Autodesk Fusion 360 part; units mm, degrees
(part 5 of 6)
  line L1119 (10, 7.0711) -> (7.0711, 10)
  line L1120 (7.0711, 10) -> (10, 12.9289)
  line L1121 (10, 12.9289) -> (12.9289, 10)
  line L1122 (12.9289, -10) -> (10, -12.9289)
  line L1123 (10, -12.9289) -> (7.0711, -10)
  line L1124 (7.0711, -10) -> (10, -7.0711)
  line L1125 (10, -7.0711) -> (12.9289, -10)
  line L1126 (2.9289, 10) -> (0, 7.0711)
  line L1127 (0, 7.0711) -> (-2.9289, 10)
  line L1128 (-2.9289, 10) -> (0, 12.9289)
  line L1129 (0, 12.9289) -> (2.9289, 10)
  line L1130 (12.9289, 0) -> (10, -2.9289)
  line L1131 (10, -2.9289) -> (7.0711, 0)
  line L1132 (7.0711, 0) -> (10, 2.9289)
  line L1133 (10, 2.9289) -> (12.9289, 0)
  line L1134 (2.9289, 0) -> (0, -2.9289)
  line L1135 (0, -2.9289) -> (-2.9289, 0)
  line L1136 (-2.9289, 0) -> (0, 2.9289)
  line L1137 (0, 2.9289) -> (2.9289, 0)
  line L1138 (2.9289, -10) -> (0, -12.9289)
  line L1139 (0, -12.9289) -> (-2.9289, -10)
  line L1140 (-2.9289, -10) -> (0, -7.0711)
  line L1141 (0, -7.0711) -> (2.9289, -10)
  line L1142 (2.9289, 40) -> (0, 37.0711)
  line L1143 (0, 37.0711) -> (-2.9289, 40)
  line L1144 (-2.9289, 40) -> (0, 42.9289)
  line L1145 (0, 42.9289) -> (2.9289, 40)
  line L1146 (42.9289, 20) -> (40, 17.0711)
  line L1147 (40, 17.0711) -> (37.0711, 20)
  line L1148 (37.0711, 20) -> (40, 22.9289)
  line L1149 (40, 22.9289) -> (42.9289, 20)
  line L1150 (-7.0711, 40) -> (-10, 37.0711)
  line L1151 (-10, 37.0711) -> (-12.9289, 40)
  line L1152 (-12.9289, 40) -> (-10, 42.9289)
  line L1153 (-10, 42.9289) -> (-7.0711, 40)
  line L1154 (42.9289, 10) -> (40, 7.0711)
  line L1155 (40, 7.0711) -> (37.0711, 10)
  line L1156 (37.0711, 10) -> (40, 12.9289)
  line L1157 (40, 12.9289) -> (42.9289, 10)
  line L1158 (42.9289, 0) -> (40, -2.9289)
  line L1159 (40, -2.9289) -> (37.0711, 0)
  line L1160 (37.0711, 0) -> (40, 2.9289)
  line L1161 (40, 2.9289) -> (42.9289, 0)
  line L1162 (42.9289, -10) -> (40, -12.9289)
  line L1163 (40, -12.9289) -> (37.0711, -10)
  line L1164 (37.0711, -10) -> (40, -7.0711)
  line L1165 (40, -7.0711) -> (42.9289, -10)
  line L1166 (42.9289, -20) -> (40, -22.9289)
  line L1167 (40, -22.9289) -> (37.0711, -20)
  line L1168 (37.0711, -20) -> (40, -17.0711)
  line L1169 (40, -17.0711) -> (42.9289, -20)
  line L1170 (42.9289, -30) -> (40, -32.9289)
  line L1171 (40, -32.9289) -> (37.0711, -30)
  line L1172 (37.0711, -30) -> (40, -27.0711)
  line L1173 (40, -27.0711) -> (42.9289, -30)
  line L1174 (42.9289, -40) -> (40, -42.9289)
  line L1175 (40, -42.9289) -> (37.0711, -40)
  line L1176 (37.0711, -40) -> (40, -37.0711)
  line L1177 (40, -37.0711) -> (42.9289, -40)
  line L1178 (32.9289, -40) -> (30, -42.9289)
  line L1179 (30, -42.9289) -> (27.0711, -40)
  line L1180 (27.0711, -40) -> (30, -37.0711)
  line L1181 (30, -37.0711) -> (32.9289, -40)
  line L1182 (22.9289, -40) -> (20, -42.9289)
  line L1183 (20, -42.9289) -> (17.0711, -40)
  line L1184 (17.0711, -40) -> (20, -37.0711)
  line L1185 (20, -37.0711) -> (22.9289, -40)
  line L1186 (12.9289, -40) -> (10, -42.9289)
  line L1187 (10, -42.9289) -> (7.0711, -40)
  line L1188 (7.0711, -40) -> (10, -37.0711)
  line L1189 (10, -37.0711) -> (12.9289, -40)
  line L1190 (2.9289, -40) -> (0, -42.9289)
  line L1191 (0, -42.9289) -> (-2.9289, -40)
  line L1192 (-2.9289, -40) -> (0, -37.0711)
  line L1193 (0, -37.0711) -> (2.9289, -40)
  line L1194 (-7.0711, -40) -> (-10, -42.9289)
  line L1195 (-10, -42.9289) -> (-12.9289, -40)
  line L1196 (-12.9289, -40) -> (-10, -37.0711)
  line L1197 (-10, -37.0711) -> (-7.0711, -40)
  line L1198 (-17.0711, -30) -> (-20, -32.9289)
  line L1199 (-20, -32.9289) -> (-22.9289, -30)
  line L1200 (-22.9289, -30) -> (-20, -27.0711)
  line L1201 (-20, -27.0711) -> (-17.0711, -30)
  line L1202 (-27.0711, -30) -> (-30, -32.9289)
  line L1203 (-30, -32.9289) -> (-32.9289, -30)
  line L1204 (-32.9289, -30) -> (-30, -27.0711)
  line L1205 (-30, -27.0711) -> (-27.0711, -30)
  line L1206 (-37.0711, -40) -> (-40, -42.9289)
  line L1207 (-40, -42.9289) -> (-42.9289, -40)
  line L1208 (-42.9289, -40) -> (-40, -37.0711)
  line L1209 (-40, -37.0711) -> (-37.0711, -40)
  line L1210 (-47.0711, -50) -> (-50, -52.9289)
  line L1211 (-50, -52.9289) -> (-52.9289, -50)
  line L1212 (-52.9289, -50) -> (-50, -47.0711)
  line L1213 (-50, -47.0711) -> (-47.0711, -50)
  line L1214 (-47.0711, -40) -> (-50, -42.9289)
  line L1215 (-50, -42.9289) -> (-52.9289, -40)
  line L1216 (-52.9289, -40) -> (-50, -37.0711)
  line L1217 (-50, -37.0711) -> (-47.0711, -40)
  line L1218 (-47.0711, -30) -> (-50, -32.9289)
  line L1219 (-50, -32.9289) -> (-52.9289, -30)
  line L1220 (-52.9289, -30) -> (-50, -27.0711)
  line L1221 (-50, -27.0711) -> (-47.0711, -30)
  line L1222 (-47.0711, -20) -> (-50, -22.9289)
  line L1223 (-50, -22.9289) -> (-52.9289, -20)
  line L1224 (-52.9289, -20) -> (-50, -17.0711)
  line L1225 (-50, -17.0711) -> (-47.0711, -20)
  line L1226 (-47.0711, -10) -> (-50, -12.9289)
  line L1227 (-50, -12.9289) -> (-52.9289, -10)
  line L1228 (-52.9289, -10) -> (-50, -7.0711)
  line L1229 (-50, -7.0711) -> (-47.0711, -10)
  line L1230 (-47.0711, 0) -> (-50, -2.9289)
  line L1231 (-50, -2.9289) -> (-52.9289, 0)
  line L1232 (-52.9289, 0) -> (-50, 2.9289)
  line L1233 (-50, 2.9289) -> (-47.0711, 0)
  line L1234 (-47.0711, 30) -> (-50, 27.0711)
  line L1235 (-50, 27.0711) -> (-52.9289, 30)
  line L1236 (-52.9289, 30) -> (-50, 32.9289)
  line L1237 (-50, 32.9289) -> (-47.0711, 30)
  line L1238 (-17.0711, -40) -> (-20, -42.9289)
  line L1239 (-20, -42.9289) -> (-22.9289, -40)
  line L1240 (-22.9289, -40) -> (-20, -37.0711)
  line L1241 (-20, -37.0711) -> (-17.0711, -40)
  line L1242 (22.9289, -50) -> (20, -52.9289)
  line L1243 (20, -52.9289) -> (17.0711, -50)
  line L1244 (17.0711, -50) -> (20, -47.0711)
  line L1245 (20, -47.0711) -> (22.9289, -50)
  line L1246 (52.9289, -40) -> (50, -42.9289)
  line L1247 (50, -42.9289) -> (47.0711, -40)
  line L1248 (47.0711, -40) -> (50, -37.0711)
  line L1249 (50, -37.0711) -> (52.9289, -40)
  line L1250 (52.9289, -50) -> (50, -52.9289)
  line L1251 (50, -52.9289) -> (47.0711, -50)
  line L1252 (47.0711, -50) -> (50, -47.0711)
  line L1253 (50, -47.0711) -> (52.9289, -50)
  line L1254 (32.9289, -50) -> (30, -52.9289)
  line L1255 (30, -52.9289) -> (27.0711, -50)
  line L1256 (27.0711, -50) -> (30, -47.0711)
  line L1257 (30, -47.0711) -> (32.9289, -50)
  line L1258 (42.9289, -50) -> (40, -52.9289)
  line L1259 (40, -52.9289) -> (37.0711, -50)
  line L1260 (37.0711, -50) -> (40, -47.0711)
  line L1261 (40, -47.0711) -> (42.9289, -50)
  line L1262 (2.9289, -50) -> (0, -52.9289)
  line L1263 (0, -52.9289) -> (-2.9289, -50)
  line L1264 (-2.9289, -50) -> (0, -47.0711)
  line L1265 (0, -47.0711) -> (2.9289, -50)
  line L1266 (12.9289, -50) -> (10, -52.9289)
  line L1267 (10, -52.9289) -> (7.0711, -50)
  line L1268 (7.0711, -50) -> (10, -47.0711)
  line L1269 (10, -47.0711) -> (12.9289, -50)
  line L1270 (-7.0711, -50) -> (-10, -52.9289)
  line L1271 (-10, -52.9289) -> (-12.9289, -50)
  line L1272 (-12.9289, -50) -> (-10, -47.0711)
  line L1273 (-10, -47.0711) -> (-7.0711, -50)
  line L1274 (-27.0711, -40) -> (-30, -42.9289)
  line L1275 (-30, -42.9289) -> (-32.9289, -40)
  line L1276 (-32.9289, -40) -> (-30, -37.0711)
  line L1277 (-30, -37.0711) -> (-27.0711, -40)
  line L1278 (-37.0711, -50) -> (-40, -52.9289)
  line L1279 (-40, -52.9289) -> (-42.9289, -50)
  line L1280 (-42.9289, -50) -> (-40, -47.0711)
  line L1281 (-40, -47.0711) -> (-37.0711, -50)
  line L1282 (-57.0711, -50) -> (-60, -52.9289)
  line L1283 (-60, -52.9289) -> (-62.9289, -50)
  line L1284 (-62.9289, -50) -> (-60, -47.0711)
  line L1285 (-60, -47.0711) -> (-57.0711, -50)
  line L1286 (-47.0711, -60) -> (-50, -62.9289)
  line L1287 (-50, -62.9289) -> (-52.9289, -60)
  line L1288 (-52.9289, -60) -> (-50, -57.0711)
  line L1289 (-50, -57.0711) -> (-47.0711, -60)
  line L1290 (52.9289, -30) -> (50, -32.9289)
  line L1291 (50, -32.9289) -> (47.0711, -30)
  line L1292 (47.0711, -30) -> (50, -27.0711)
  line L1293 (50, -27.0711) -> (52.9289, -30)
  line L1294 (52.9289, -20) -> (50, -22.9289)
  line L1295 (50, -22.9289) -> (47.0711, -20)
  line L1296 (47.0711, -20) -> (50, -17.0711)
  line L1297 (50, -17.0711) -> (52.9289, -20)
  line L1298 (52.9289, -10) -> (50, -12.9289)
  line L1299 (50, -12.9289) -> (47.0711, -10)
  line L1300 (47.0711, -10) -> (50, -7.0711)
  line L1301 (50, -7.0711) -> (52.9289, -10)
  line L1302 (52.9289, 0) -> (50, -2.9289)
  line L1303 (50, -2.9289) -> (47.0711, 0)
  line L1304 (47.0711, 0) -> (50, 2.9289)
  line L1305 (50, 2.9289) -> (52.9289, 0)
  line L1306 (52.9289, 10) -> (50, 7.0711)
  line L1307 (50, 7.0711) -> (47.0711, 10)
  line L1308 (47.0711, 10) -> (50, 12.9289)
  line L1309 (50, 12.9289) -> (52.9289, 10)
  line L1310 (52.9289, 20) -> (50, 17.0711)
  line L1311 (50, 17.0711) -> (47.0711, 20)
  line L1312 (47.0711, 20) -> (50, 22.9289)
  line L1313 (50, 22.9289) -> (52.9289, 20)
  line L1314 (2.9289, 50) -> (0, 47.0711)
  line L1315 (0, 47.0711) -> (-2.9289, 50)
  line L1316 (-2.9289, 50) -> (0, 52.9289)
  line L1317 (0, 52.9289) -> (2.9289, 50)
  line L1318 (-7.0711, 50) -> (-10, 47.0711)
  line L1319 (-10, 47.0711) -> (-12.9289, 50)
  line L1320 (-12.9289, 50) -> (-10, 52.9289)
  line L1321 (-10, 52.9289) -> (-7.0711, 50)
  line L1322 (-17.0711, 50) -> (-20, 47.0711)
  line L1323 (-20, 47.0711) -> (-22.9289, 50)
  line L1324 (-22.9289, 50) -> (-20, 52.9289)
  line L1325 (-20, 52.9289) -> (-17.0711, 50)
  line L1326 (-27.0711, 50) -> (-30, 47.0711)
  line L1327 (-30, 47.0711) -> (-32.9289, 50)
  line L1328 (-32.9289, 50) -> (-30, 52.9289)
  line L1329 (-30, 52.9289) -> (-27.0711, 50)
  line L1330 (-37.0711, 50) -> (-40, 47.0711)
  line L1331 (-40, 47.0711) -> (-42.9289, 50)
  line L1332 (-42.9289, 50) -> (-40, 52.9289)
  line L1333 (-40, 52.9289) -> (-37.0711, 50)
  line L1334 (-47.0711, 50) -> (-50, 47.0711)
  line L1335 (-50, 47.0711) -> (-52.9289, 50)
  line L1336 (-52.9289, 50) -> (-50, 52.9289)
  line L1337 (-50, 52.9289) -> (-47.0711, 50)
  line L1338 (-47.0711, 40) -> (-50, 37.0711)
  line L1339 (-50, 37.0711) -> (-52.9289, 40)
  line L1340 (-52.9289, 40) -> (-50, 42.9289)
  line L1341 (-50, 42.9289) -> (-47.0711, 40)
  line L1342 (-47.0711, 10) -> (-50, 7.0711)
  line L1343 (-50, 7.0711) -> (-52.9289, 10)
  line L1344 (-52.9289, 10) -> (-50, 12.9289)
  line L1345 (-50, 12.9289) -> (-47.0711, 10)
  line L1346 (-47.0711, 20) -> (-50, 17.0711)
  line L1347 (-50, 17.0711) -> (-52.9289, 20)
  line L1348 (-52.9289, 20) -> (-50, 22.9289)
  line L1349 (-50, 22.9289) -> (-47.0711, 20)
  line L1350 (-39, -6.6569) -> (-39, -3.3431)
  line L1351 (-39, -3.3431) -> (-36.6569, -1)
  line L1352 (-36.6569, -1) -> (-33.3431, -1)
  line L1353 (-33.3431, -1) -> (-31, -3.3431)
  line L1354 (-31, -3.3431) -> (-31, -6.6569)
  line L1355 (-31, -6.6569) -> (-33.3431, -9)
  line L1356 (-33.3431, -9) -> (-36.6569, -9)
  line L1357 (-36.6569, -9) -> (-39, -6.6569)
  line L1358 (-49, -6.6569) -> (-49, -3.3431)
  line L1359 (-49, -3.3431) -> (-46.6569, -1)
  line L1360 (-46.6569, -1) -> (-43.3431, -1)
  line L1361 (-43.3431, -1) -> (-41, -3.3431)
  line L1362 (-41, -3.3431) -> (-41, -6.6569)
  line L1363 (-41, -6.6569) -> (-43.3431, -9)
  line L1364 (-43.3431, -9) -> (-46.6569, -9)
  line L1365 (-46.6569, -9) -> (-49, -6.6569)
  line L1366 (-29, -6.6569) -> (-29, -3.3431)
  line L1367 (-29, -3.3431) -> (-26.6569, -1)
  line L1368 (-26.6569, -1) -> (-23.3431, -1)
  line L1369 (-23.3431, -1) -> (-21, -3.3431)
  line L1370 (-21, -3.3431) -> (-21, -6.6569)
  line L1371 (-21, -6.6569) -> (-23.3431, -9)
  line L1372 (-23.3431, -9) -> (-26.6569, -9)
  line L1373 (-26.6569, -9) -> (-29, -6.6569)
  line L1374 (-59, -6.6569) -> (-59, -3.3431)
  line L1375 (-59, -3.3431) -> (-56.6569, -1)
  line L1376 (-56.6569, -1) -> (-53.3431, -1)
  line L1377 (-53.3431, -1) -> (-51, -3.3431)
  line L1378 (-51, -3.3431) -> (-51, -6.6569)
  line L1379 (-51, -6.6569) -> (-53.3431, -9)
  line L1380 (-53.3431, -9) -> (-56.6569, -9)
  line L1381 (-56.6569, -9) -> (-59, -6.6569)
  line L1382 (-69, -6.6569) -> (-69, -3.3431)
  line L1383 (-69, -3.3431) -> (-66.6569, -1)
  line L1384 (-66.6569, -1) -> (-63.3431, -1)
  line L1385 (-63.3431, -1) -> (-61, -3.3431)
  line L1386 (-61, -3.3431) -> (-61, -6.6569)
  line L1387 (-61, -6.6569) -> (-63.3431, -9)
  line L1388 (-63.3431, -9) -> (-66.6569, -9)
  line L1389 (-66.6569, -9) -> (-69, -6.6569)
  line L1390 (61, -16.6569) -> (61, -13.3431)
  line L1391 (61, -13.3431) -> (63.3431, -11)
  line L1392 (63.3431, -11) -> (66.6569, -11)
  line L1393 (66.6569, -11) -> (69, -13.3431)
  line L1394 (69, -13.3431) -> (69, -16.6569)
  line L1395 (69, -16.6569) -> (66.6569, -19)
  line L1396 (66.6569, -19) -> (63.3431, -19)
  line L1397 (63.3431, -19) -> (61, -16.6569)
  line L1398 (-19, -6.6569) -> (-19, -3.3431)
  line L1399 (-19, -3.3431) -> (-16.6569, -1)
  line L1400 (-16.6569, -1) -> (-13.3431, -1)
  line L1401 (-13.3431, -1) -> (-11, -3.3431)
  line L1402 (-11, -3.3431) -> (-11, -6.6569)
  line L1403 (-11, -6.6569) -> (-13.3431, -9)
  line L1404 (-13.3431, -9) -> (-16.6569, -9)
  line L1405 (-16.6569, -9) -> (-19, -6.6569)
  line L1406 (51, -16.6569) -> (51, -13.3431)
  line L1407 (51, -13.3431) -> (53.3431, -11)
  line L1408 (53.3431, -11) -> (56.6569, -11)
  line L1409 (56.6569, -11) -> (59, -13.3431)
  line L1410 (59, -13.3431) -> (59, -16.6569)
  line L1411 (59, -16.6569) -> (56.6569, -19)
  line L1412 (56.6569, -19) -> (53.3431, -19)
  line L1413 (53.3431, -19) -> (51, -16.6569)
  line L1414 (41, -16.6569) -> (41, -13.3431)
  line L1415 (41, -13.3431) -> (43.3431, -11)
  line L1416 (43.3431, -11) -> (46.6569, -11)
  line L1417 (46.6569, -11) -> (49, -13.3431)
  line L1418 (49, -13.3431) -> (49, -16.6569)
  line L1419 (49, -16.6569) -> (46.6569, -19)
  line L1420 (46.6569, -19) -> (43.3431, -19)
  line L1421 (43.3431, -19) -> (41, -16.6569)
  line L1422 (-9, -6.6569) -> (-9, -3.3431)
  line L1423 (-9, -3.3431) -> (-6.6569, -1)
  line L1424 (-6.6569, -1) -> (-3.3431, -1)
  line L1425 (-3.3431, -1) -> (-1, -3.3431)
  line L1426 (-1, -3.3431) -> (-1, -6.6569)
  line L1427 (-1, -6.6569) -> (-3.3431, -9)
  line L1428 (-3.3431, -9) -> (-6.6569, -9)
  line L1429 (-6.6569, -9) -> (-9, -6.6569)
  line L1430 (-9, 13.3431) -> (-9, 16.6569)
  line L1431 (-9, 16.6569) -> (-6.6569, 19)
  line L1432 (-6.6569, 19) -> (-3.3431, 19)
  line L1433 (-3.3431, 19) -> (-1, 16.6569)
  line L1434 (-1, 16.6569) -> (-1, 13.3431)
  line L1435 (-1, 13.3431) -> (-3.3431, 11)
  line L1436 (-3.3431, 11) -> (-6.6569, 11)
  line L1437 (-6.6569, 11) -> (-9, 13.3431)
  line L1438 (-39, 13.3431) -> (-39, 16.6569)
  line L1439 (-39, 16.6569) -> (-36.6569, 19)
  line L1440 (-36.6569, 19) -> (-33.3431, 19)
  line L1441 (-33.3431, 19) -> (-31, 16.6569)
  line L1442 (-31, 16.6569) -> (-31, 13.3431)
  line L1443 (-31, 13.3431) -> (-33.3431, 11)
  line L1444 (-33.3431, 11) -> (-36.6569, 11)
  line L1445 (-36.6569, 11) -> (-39, 13.3431)
  line L1446 (1, 13.3431) -> (1, 16.6569)
  line L1447 (1, 16.6569) -> (3.3431, 19)
  line L1448 (3.3431, 19) -> (6.6569, 19)
  line L1449 (6.6569, 19) -> (9, 16.6569)
  line L1450 (9, 16.6569) -> (9, 13.3431)
  line L1451 (9, 13.3431) -> (6.6569, 11)
  line L1452 (6.6569, 11) -> (3.3431, 11)
  line L1453 (3.3431, 11) -> (1, 13.3431)
  line L1454 (31, 13.3431) -> (31, 16.6569)
  line L1455 (31, 16.6569) -> (33.3431, 19)
  line L1456 (33.3431, 19) -> (36.6569, 19)
  line L1457 (36.6569, 19) -> (39, 16.6569)
  line L1458 (39, 16.6569) -> (39, 13.3431)
  line L1459 (39, 13.3431) -> (36.6569, 11)
  line L1460 (36.6569, 11) -> (33.3431, 11)
  line L1461 (33.3431, 11) -> (31, 13.3431)
  line L1462 (11, 13.3431) -> (11, 16.6569)
  line L1463 (11, 16.6569) -> (13.3431, 19)
  line L1464 (13.3431, 19) -> (16.6569, 19)
  line L1465 (16.6569, 19) -> (19, 16.6569)
  line L1466 (19, 16.6569) -> (19, 13.3431)
  line L1467 (19, 13.3431) -> (16.6569, 11)
  line L1468 (16.6569, 11) -> (13.3431, 11)
  line L1469 (13.3431, 11) -> (11, 13.3431)
  line L1470 (21, 13.3431) -> (21, 16.6569)
  line L1471 (21, 16.6569) -> (23.3431, 19)
  line L1472 (23.3431, 19) -> (26.6569, 19)
  line L1473 (26.6569, 19) -> (29, 16.6569)
  line L1474 (29, 16.6569) -> (29, 13.3431)
  line L1475 (29, 13.3431) -> (26.6569, 11)
  line L1476 (26.6569, 11) -> (23.3431, 11)
  line L1477 (23.3431, 11) -> (21, 13.3431)
  line L1478 (-39, 63.3431) -> (-39, 66.6569)
  line L1479 (-39, 66.6569) -> (-36.6569, 69)
  line L1480 (-36.6569, 69) -> (-33.3431, 69)
  line L1481 (-33.3431, 69) -> (-31, 66.6569)
  line L1482 (-31, 66.6569) -> (-31, 63.3431)
  line L1483 (-31, 63.3431) -> (-33.3431, 61)
  line L1484 (-33.3431, 61) -> (-36.6569, 61)
  line L1485 (-36.6569, 61) -> (-39, 63.3431)
  line L1486 (-49, 63.3431) -> (-49, 66.6569)
  line L1487 (-49, 66.6569) -> (-46.6569, 69)
  line L1488 (-46.6569, 69) -> (-43.3431, 69)
  line L1489 (-43.3431, 69) -> (-41, 66.6569)
  line L1490 (-41, 66.6569) -> (-41, 63.3431)
  line L1491 (-41, 63.3431) -> (-43.3431, 61)
  line L1492 (-43.3431, 61) -> (-46.6569, 61)
  line L1493 (-46.6569, 61) -> (-49, 63.3431)
  line L1494 (51, 63.3431) -> (51, 66.6569)
  line L1495 (51, 66.6569) -> (53.3431, 69)
  line L1496 (53.3431, 69) -> (56.6569, 69)
  line L1497 (56.6569, 69) -> (59, 66.6569)
  line L1498 (59, 66.6569) -> (59, 63.3431)
  line L1499 (59, 63.3431) -> (56.6569, 61)
  line L1500 (56.6569, 61) -> (53.3431, 61)
  line L1501 (53.3431, 61) -> (51, 63.3431)
  line L1502 (31, 63.3431) -> (31, 66.6569)
  line L1503 (31, 66.6569) -> (33.3431, 69)
  line L1504 (33.3431, 69) -> (36.6569, 69)
  line L1505 (36.6569, 69) -> (39, 66.6569)
  line L1506 (39, 66.6569) -> (39, 63.3431)
  line L1507 (39, 63.3431) -> (36.6569, 61)
  line L1508 (36.6569, 61) -> (33.3431, 61)
  line L1509 (33.3431, 61) -> (31, 63.3431)
  line L1510 (11, 63.3431) -> (11, 66.6569)
  line L1511 (11, 66.6569) -> (13.3431, 69)
  line L1512 (13.3431, 69) -> (16.6569, 69)
  line L1513 (16.6569, 69) -> (19, 66.6569)
  line L1514 (19, 66.6569) -> (19, 63.3431)
  line L1515 (19, 63.3431) -> (16.6569, 61)
  line L1516 (16.6569, 61) -> (13.3431, 61)
  line L1517 (13.3431, 61) -> (11, 63.3431)
  line L1518 (61, 63.3431) -> (61, 66.6569)
  line L1519 (61, 66.6569) -> (63.3431, 69)
  line L1520 (63.3431, 69) -> (66.6569, 69)
  line L1521 (66.6569, 69) -> (69, 66.6569)
  line L1522 (69, 66.6569) -> (69, 63.3431)
  line L1523 (69, 63.3431) -> (66.6569, 61)
  line L1524 (66.6569, 61) -> (63.3431, 61)
  line L1525 (63.3431, 61) -> (61, 63.3431)
  line L1526 (41, 63.3431) -> (41, 66.6569)
  line L1527 (41, 66.6569) -> (43.3431, 69)
  line L1528 (43.3431, 69) -> (46.6569, 69)
  line L1529 (46.6569, 69) -> (49, 66.6569)
  line L1530 (49, 66.6569) -> (49, 63.3431)
  line L1531 (49, 63.3431) -> (46.6569, 61)
  line L1532 (46.6569, 61) -> (43.3431, 61)
  line L1533 (43.3431, 61) -> (41, 63.3431)
  line L1534 (-9, 63.3431) -> (-9, 66.6569)
  line L1535 (-9, 66.6569) -> (-6.6569, 69)
  line L1536 (-6.6569, 69) -> (-3.3431, 69)
  line L1537 (-3.3431, 69) -> (-1, 66.6569)
  line L1538 (-1, 66.6569) -> (-1, 63.3431)
  line L1539 (-1, 63.3431) -> (-3.3431, 61)
  line L1540 (-3.3431, 61) -> (-6.6569, 61)
  line L1541 (-6.6569, 61) -> (-9, 63.3431)
  line L1542 (21, 63.3431) -> (21, 66.6569)
  line L1543 (21, 66.6569) -> (23.3431, 69)
  line L1544 (23.3431, 69) -> (26.6569, 69)
  line L1545 (26.6569, 69) -> (29, 66.6569)
  line L1546 (29, 66.6569) -> (29, 63.3431)
  line L1547 (29, 63.3431) -> (26.6569, 61)
  line L1548 (26.6569, 61) -> (23.3431, 61)
  line L1549 (23.3431, 61) -> (21, 63.3431)
  line L1550 (1, 63.3431) -> (1, 66.6569)
  line L1551 (1, 66.6569) -> (3.3431, 69)
  line L1552 (3.3431, 69) -> (6.6569, 69)
  line L1553 (6.6569, 69) -> (9, 66.6569)
  line L1554 (9, 66.6569) -> (9, 63.3431)
  line L1555 (9, 63.3431) -> (6.6569, 61)
  line L1556 (6.6569, 61) -> (3.3431, 61)
  line L1557 (3.3431, 61) -> (1, 63.3431)
  line L1558 (-29, 63.3431) -> (-29, 66.6569)
  line L1559 (-29, 66.6569) -> (-26.6569, 69)
  line L1560 (-26.6569, 69) -> (-23.3431, 69)
  line L1561 (-23.3431, 69) -> (-21, 66.6569)
  line L1562 (-21, 66.6569) -> (-21, 63.3431)
  line L1563 (-21, 63.3431) -> (-23.3431, 61)
  line L1564 (-23.3431, 61) -> (-26.6569, 61)
  line L1565 (-26.6569, 61) -> (-29, 63.3431)
  line L1566 (-19, 63.3431) -> (-19, 66.6569)
  line L1567 (-19, 66.6569) -> (-16.6569, 69)
  line L1568 (-16.6569, 69) -> (-13.3431, 69)
  line L1569 (-13.3431, 69) -> (-11, 66.6569)
  line L1570 (-11, 66.6569) -> (-11, 63.3431)
  line L1571 (-11, 63.3431) -> (-13.3431, 61)
  line L1572 (-13.3431, 61) -> (-16.6569, 61)
  line L1573 (-16.6569, 61) -> (-19, 63.3431)
  line L1574 (51, -26.6569) -> (51, -23.3431)
  line L1575 (51, -23.3431) -> (53.3431, -21)
  line L1576 (53.3431, -21) -> (56.6569, -21)
  line L1577 (56.6569, -21) -> (59, -23.3431)
  line L1578 (59, -23.3431) -> (59, -26.6569)
  line L1579 (59, -26.6569) -> (56.6569, -29)
  line L1580 (56.6569, -29) -> (53.3431, -29)
  line L1581 (53.3431, -29) -> (51, -26.6569)
  line L1582 (-69, -16.6569) -> (-69, -13.3431)
  line L1583 (-69, -13.3431) -> (-66.6569, -11)
  line L1584 (-66.6569, -11) -> (-63.3431, -11)
  line L1585 (-63.3431, -11) -> (-61, -13.3431)
  line L1586 (-61, -13.3431) -> (-61, -16.6569)
  line L1587 (-61, -16.6569) -> (-63.3431, -19)
  line L1588 (-63.3431, -19) -> (-66.6569, -19)
  line L1589 (-66.6569, -19) -> (-69, -16.6569)
  line L1590 (-59, -16.6569) -> (-59, -13.3431)
  line L1591 (-59, -13.3431) -> (-56.6569, -11)
  line L1592 (-56.6569, -11) -> (-53.3431, -11)
  line L1593 (-53.3431, -11) -> (-51, -13.3431)
  line L1594 (-51, -13.3431) -> (-51, -16.6569)
  line L1595 (-51, -16.6569) -> (-53.3431, -19)
  line L1596 (-53.3431, -19) -> (-56.6569, -19)
  line L1597 (-56.6569, -19) -> (-59, -16.6569)
  line L1598 (-49, -16.6569) -> (-49, -13.3431)
  line L1599 (-49, -13.3431) -> (-46.6569, -11)
  line L1600 (-46.6569, -11) -> (-43.3431, -11)
  line L1601 (-43.3431, -11) -> (-41, -13.3431)
  line L1602 (-41, -13.3431) -> (-41, -16.6569)
  line L1603 (-41, -16.6569) -> (-43.3431, -19)
  line L1604 (-43.3431, -19) -> (-46.6569, -19)
  line L1605 (-46.6569, -19) -> (-49, -16.6569)
  line L1606 (-29, -16.6569) -> (-29, -13.3431)
  line L1607 (-29, -13.3431) -> (-26.6569, -11)
  line L1608 (-26.6569, -11) -> (-23.3431, -11)
  line L1609 (-23.3431, -11) -> (-21, -13.3431)
  line L1610 (-21, -13.3431) -> (-21, -16.6569)
  line L1611 (-21, -16.6569) -> (-23.3431, -19)
  line L1612 (-23.3431, -19) -> (-26.6569, -19)
  line L1613 (-26.6569, -19) -> (-29, -16.6569)
  line L1614 (-9, -16.6569) -> (-9, -13.3431)
  line L1615 (-9, -13.3431) -> (-6.6569, -11)
  line L1616 (-6.6569, -11) -> (-3.3431, -11)
  line L1617 (-3.3431, -11) -> (-1, -13.3431)
  line L1618 (-1, -13.3431) -> (-1, -16.6569)
  line L1619 (-1, -16.6569) -> (-3.3431, -19)
  line L1620 (-3.3431, -19) -> (-6.6569, -19)
  line L1621 (-6.6569, -19) -> (-9, -16.6569)
  line L1622 (1, -36.6569) -> (1, -33.3431)
  line L1623 (1, -33.3431) -> (3.3431, -31)
  line L1624 (3.3431, -31) -> (6.6569, -31)
  line L1625 (6.6569, -31) -> (9, -33.3431)
  line L1626 (9, -33.3431) -> (9, -36.6569)
  line L1627 (9, -36.6569) -> (6.6569, -39)
  line L1628 (6.6569, -39) -> (3.3431, -39)
  line L1629 (3.3431, -39) -> (1, -36.6569)
  line L1630 (-9, -26.6569) -> (-9, -23.3431)
  line L1631 (-9, -23.3431) -> (-6.6569, -21)
  line L1632 (-6.6569, -21) -> (-3.3431, -21)
  line L1633 (-3.3431, -21) -> (-1, -23.3431)
  line L1634 (-1, -23.3431) -> (-1, -26.6569)
  line L1635 (-1, -26.6569) -> (-3.3431, -29)
  line L1636 (-3.3431, -29) -> (-6.6569, -29)
  line L1637 (-6.6569, -29) -> (-9, -26.6569)
  line L1638 (1, -26.6569) -> (1, -23.3431)
  line L1639 (1, -23.3431) -> (3.3431, -21)
  line L1640 (3.3431, -21) -> (6.6569, -21)
  line L1641 (6.6569, -21) -> (9, -23.3431)
  line L1642 (9, -23.3431) -> (9, -26.6569)
  line L1643 (9, -26.6569) -> (6.6569, -29)
  line L1644 (6.6569, -29) -> (3.3431, -29)
  line L1645 (3.3431, -29) -> (1, -26.6569)
  line L1646 (-49, -36.6569) -> (-49, -33.3431)
  line L1647 (-49, -33.3431) -> (-46.6569, -31)
  line L1648 (-46.6569, -31) -> (-43.3431, -31)
  line L1649 (-43.3431, -31) -> (-41, -33.3431)
  line L1650 (-41, -33.3431) -> (-41, -36.6569)
  line L1651 (-41, -36.6569) -> (-43.3431, -39)
  line L1652 (-43.3431, -39) -> (-46.6569, -39)
  line L1653 (-46.6569, -39) -> (-49, -36.6569)
  line L1654 (-9, -36.6569) -> (-9, -33.3431)
  line L1655 (-9, -33.3431) -> (-6.6569, -31)
  line L1656 (-6.6569, -31) -> (-3.3431, -31)
  line L1657 (-3.3431, -31) -> (-1, -33.3431)
  line L1658 (-1, -33.3431) -> (-1, -36.6569)
  line L1659 (-1, -36.6569) -> (-3.3431, -39)
  line L1660 (-3.3431, -39) -> (-6.6569, -39)
  line L1661 (-6.6569, -39) -> (-9, -36.6569)
  line L1662 (-19, -36.6569) -> (-19, -33.3431)
  line L1663 (-19, -33.3431) -> (-16.6569, -31)
  line L1664 (-16.6569, -31) -> (-13.3431, -31)
  line L1665 (-13.3431, -31) -> (-11, -33.3431)
  line L1666 (-11, -33.3431) -> (-11, -36.6569)
  line L1667 (-11, -36.6569) -> (-13.3431, -39)
  line L1668 (-13.3431, -39) -> (-16.6569, -39)
  line L1669 (-16.6569, -39) -> (-19, -36.6569)
  line L1670 (-29, -36.6569) -> (-29, -33.3431)
  line L1671 (-29, -33.3431) -> (-26.6569, -31)
  line L1672 (-26.6569, -31) -> (-23.3431, -31)
  line L1673 (-23.3431, -31) -> (-21, -33.3431)
  line L1674 (-21, -33.3431) -> (-21, -36.6569)
  line L1675 (-21, -36.6569) -> (-23.3431, -39)
  line L1676 (-23.3431, -39) -> (-26.6569, -39)
  line L1677 (-26.6569, -39) -> (-29, -36.6569)
  line L1678 (-39, -36.6569) -> (-39, -33.3431)
  line L1679 (-39, -33.3431) -> (-36.6569, -31)
  line L1680 (-36.6569, -31) -> (-33.3431, -31)
  line L1681 (-33.3431, -31) -> (-31, -33.3431)
  line L1682 (-31, -33.3431) -> (-31, -36.6569)
  line L1683 (-31, -36.6569) -> (-33.3431, -39)
  line L1684 (-33.3431, -39) -> (-36.6569, -39)
  line L1685 (-36.6569, -39) -> (-39, -36.6569)
  line L1686 (31, -26.6569) -> (31, -23.3431)
  line L1687 (31, -23.3431) -> (33.3431, -21)
  line L1688 (33.3431, -21) -> (36.6569, -21)
  line L1689 (36.6569, -21) -> (39, -23.3431)
  line L1690 (39, -23.3431) -> (39, -26.6569)
  line L1691 (39, -26.6569) -> (36.6569, -29)
  line L1692 (36.6569, -29) -> (33.3431, -29)
  line L1693 (33.3431, -29) -> (31, -26.6569)
  line L1694 (21, -26.6569) -> (21, -23.3431)
  line L1695 (21, -23.3431) -> (23.3431, -21)
  line L1696 (23.3431, -21) -> (26.6569, -21)
  line L1697 (26.6569, -21) -> (29, -23.3431)
  line L1698 (29, -23.3431) -> (29, -26.6569)
  line L1699 (29, -26.6569) -> (26.6569, -29)
  line L1700 (26.6569, -29) -> (23.3431, -29)
  line L1701 (23.3431, -29) -> (21, -26.6569)
  line L1702 (11, -26.6569) -> (11, -23.3431)
  line L1703 (11, -23.3431) -> (13.3431, -21)
  line L1704 (13.3431, -21) -> (16.6569, -21)
  line L1705 (16.6569, -21) -> (19, -23.3431)
  line L1706 (19, -23.3431) -> (19, -26.6569)
  line L1707 (19, -26.6569) -> (16.6569, -29)
  line L1708 (16.6569, -29) -> (13.3431, -29)
  line L1709 (13.3431, -29) -> (11, -26.6569)
  line L1710 (-59, -36.6569) -> (-59, -33.3431)
  line L1711 (-59, -33.3431) -> (-56.6569, -31)
  line L1712 (-56.6569, -31) -> (-53.3431, -31)
  line L1713 (-53.3431, -31) -> (-51, -33.3431)
  line L1714 (-51, -33.3431) -> (-51, -36.6569)
  line L1715 (-51, -36.6569) -> (-53.3431, -39)
  line L1716 (-53.3431, -39) -> (-56.6569, -39)
  line L1717 (-56.6569, -39) -> (-59, -36.6569)
  line L1718 (-69, -36.6569) -> (-69, -33.3431)
  line L1719 (-69, -33.3431) -> (-66.6569, -31)
  line L1720 (-66.6569, -31) -> (-63.3431, -31)
  line L1721 (-63.3431, -31) -> (-61, -33.3431)
  line L1722 (-61, -33.3431) -> (-61, -36.6569)
  line L1723 (-61, -36.6569) -> (-63.3431, -39)
  line L1724 (-63.3431, -39) -> (-66.6569, -39)
  line L1725 (-66.6569, -39) -> (-69, -36.6569)
  line L1726 (1, -46.6569) -> (1, -43.3431)
  line L1727 (1, -43.3431) -> (3.3431, -41)
  line L1728 (3.3431, -41) -> (6.6569, -41)
  line L1729 (6.6569, -41) -> (9, -43.3431)
  line L1730 (9, -43.3431) -> (9, -46.6569)
  line L1731 (9, -46.6569) -> (6.6569, -49)
  line L1732 (6.6569, -49) -> (3.3431, -49)
  line L1733 (3.3431, -49) -> (1, -46.6569)
  line L1734 (-9, -46.6569) -> (-9, -43.3431)
  line L1735 (-9, -43.3431) -> (-6.6569, -41)
  line L1736 (-6.6569, -41) -> (-3.3431, -41)
  line L1737 (-3.3431, -41) -> (-1, -43.3431)
  line L1738 (-1, -43.3431) -> (-1, -46.6569)
  line L1739 (-1, -46.6569) -> (-3.3431, -49)
  line L1740 (-3.3431, -49) -> (-6.6569, -49)
  line L1741 (-6.6569, -49) -> (-9, -46.6569)
  line L1742 (11, -36.6569) -> (11, -33.3431)
  line L1743 (11, -33.3431) -> (13.3431, -31)
  line L1744 (13.3431, -31) -> (16.6569, -31)
  line L1745 (16.6569, -31) -> (19, -33.3431)
  line L1746 (19, -33.3431) -> (19, -36.6569)
  line L1747 (19, -36.6569) -> (16.6569, -39)
  line L1748 (16.6569, -39) -> (13.3431, -39)
  line L1749 (13.3431, -39) -> (11, -36.6569)
  line L1750 (21, -36.6569) -> (21, -33.3431)
  line L1751 (21, -33.3431) -> (23.3431, -31)
  line L1752 (23.3431, -31) -> (26.6569, -31)
  line L1753 (26.6569, -31) -> (29, -33.3431)
  line L1754 (29, -33.3431) -> (29, -36.6569)
  line L1755 (29, -36.6569) -> (26.6569, -39)
  line L1756 (26.6569, -39) -> (23.3431, -39)
  line L1757 (23.3431, -39) -> (21, -36.6569)
  line L1758 (61, -46.6569) -> (61, -43.3431)
  line L1759 (61, -43.3431) -> (63.3431, -41)
  line L1760 (63.3431, -41) -> (66.6569, -41)
  line L1761 (66.6569, -41) -> (69, -43.3431)
  line L1762 (69, -43.3431) -> (69, -46.6569)
  line L1763 (69, -46.6569) -> (66.6569, -49)
  line L1764 (66.6569, -49) -> (63.3431, -49)
  line L1765 (63.3431, -49) -> (61, -46.6569)
  line L1766 (51, -46.6569) -> (51, -43.3431)
  line L1767 (51, -43.3431) -> (53.3431, -41)
  line L1768 (53.3431, -41) -> (56.6569, -41)
  line L1769 (56.6569, -41) -> (59, -43.3431)
  line L1770 (59, -43.3431) -> (59, -46.6569)
  line L1771 (59, -46.6569) -> (56.6569, -49)
  line L1772 (56.6569, -49) -> (53.3431, -49)
  line L1773 (53.3431, -49) -> (51, -46.6569)
  line L1774 (41, -46.6569) -> (41, -43.3431)
  line L1775 (41, -43.3431) -> (43.3431, -41)
  line L1776 (43.3431, -41) -> (46.6569, -41)
  line L1777 (46.6569, -41) -> (49, -43.3431)
  line L1778 (49, -43.3431) -> (49, -46.6569)
  line L1779 (49, -46.6569) -> (46.6569, -49)
  line L1780 (46.6569, -49) -> (43.3431, -49)
  line L1781 (43.3431, -49) -> (41, -46.6569)
  line L1782 (31, -46.6569) -> (31, -43.3431)
  line L1783 (31, -43.3431) -> (33.3431, -41)
  line L1784 (33.3431, -41) -> (36.6569, -41)
  line L1785 (36.6569, -41) -> (39, -43.3431)
  line L1786 (39, -43.3431) -> (39, -46.6569)
  line L1787 (39, -46.6569) -> (36.6569, -49)
  line L1788 (36.6569, -49) -> (33.3431, -49)
  line L1789 (33.3431, -49) -> (31, -46.6569)
  line L1790 (11, -46.6569) -> (11, -43.3431)
  line L1791 (11, -43.3431) -> (13.3431, -41)
  line L1792 (13.3431, -41) -> (16.6569, -41)
  line L1793 (16.6569, -41) -> (19, -43.3431)
  line L1794 (19, -43.3431) -> (19, -46.6569)
  line L1795 (19, -46.6569) -> (16.6569, -49)
  line L1796 (16.6569, -49) -> (13.3431, -49)
  line L1797 (13.3431, -49) -> (11, -46.6569)
  line L1798 (21, -46.6569) -> (21, -43.3431)
  line L1799 (21, -43.3431) -> (23.3431, -41)
  line L1800 (23.3431, -41) -> (26.6569, -41)
  line L1801 (26.6569, -41) -> (29, -43.3431)
  line L1802 (29, -43.3431) -> (29, -46.6569)
  line L1803 (29, -46.6569) -> (26.6569, -49)
  line L1804 (26.6569, -49) -> (23.3431, -49)
  line L1805 (23.3431, -49) -> (21, -46.6569)
  line L1806 (31, -36.6569) -> (31, -33.3431)
  line L1807 (31, -33.3431) -> (33.3431, -31)
  line L1808 (33.3431, -31) -> (36.6569, -31)
  line L1809 (36.6569, -31) -> (39, -33.3431)
  line L1810 (39, -33.3431) -> (39, -36.6569)
  line L1811 (39, -36.6569) -> (36.6569, -39)
  line L1812 (36.6569, -39) -> (33.3431, -39)
  line L1813 (33.3431, -39) -> (31, -36.6569)
  line L1814 (41, -36.6569) -> (41, -33.3431)
  line L1815 (41, -33.3431) -> (43.3431, -31)
  line L1816 (43.3431, -31) -> (46.6569, -31)
  line L1817 (46.6569, -31) -> (49, -33.3431)
  line L1818 (49, -33.3431) -> (49, -36.6569)
  line L1819 (49, -36.6569) -> (46.6569, -39)
  line L1820 (46.6569, -39) -> (43.3431, -39)
  line L1821 (43.3431, -39) -> (41, -36.6569)
  line L1822 (51, -36.6569) -> (51, -33.3431)
  line L1823 (51, -33.3431) -> (53.3431, -31)
  line L1824 (53.3431, -31) -> (56.6569, -31)
  line L1825 (56.6569, -31) -> (59, -33.3431)
  line L1826 (59, -33.3431) -> (59, -36.6569)
  line L1827 (59, -36.6569) -> (56.6569, -39)
  line L1828 (56.6569, -39) -> (53.3431, -39)
  line L1829 (53.3431, -39) -> (51, -36.6569)
  line L1830 (61, -36.6569) -> (61, -33.3431)
  line L1831 (61, -33.3431) -> (63.3431, -31)
  line L1832 (63.3431, -31) -> (66.6569, -31)
  line L1833 (66.6569, -31) -> (69, -33.3431)
  line L1834 (69, -33.3431) -> (69, -36.6569)
  line L1835 (69, -36.6569) -> (66.6569, -39)
  line L1836 (66.6569, -39) -> (63.3431, -39)
  line L1837 (63.3431, -39) -> (61, -36.6569)
  line L1838 (-69, -26.6569) -> (-69, -23.3431)
  line L1839 (-69, -23.3431) -> (-66.6569, -21)
  line L1840 (-66.6569, -21) -> (-63.3431, -21)
  line L1841 (-63.3431, -21) -> (-61, -23.3431)
  line L1842 (-61, -23.3431) -> (-61, -26.6569)
  line L1843 (-61, -26.6569) -> (-63.3431, -29)
  line L1844 (-63.3431, -29) -> (-66.6569, -29)
  line L1845 (-66.6569, -29) -> (-69, -26.6569)
  line L1846 (21, -16.6569) -> (21, -13.3431)
  line L1847 (21, -13.3431) -> (23.3431, -11)
  line L1848 (23.3431, -11) -> (26.6569, -11)
  line L1849 (26.6569, -11) -> (29, -13.3431)
  line L1850 (29, -13.3431) -> (29, -16.6569)
  line L1851 (29, -16.6569) -> (26.6569, -19)
  line L1852 (26.6569, -19) -> (23.3431, -19)
  line L1853 (23.3431, -19) -> (21, -16.6569)
  line L1854 (31, -16.6569) -> (31, -13.3431)
  line L1855 (31, -13.3431) -> (33.3431, -11)
  line L1856 (33.3431, -11) -> (36.6569, -11)
  line L1857 (36.6569, -11) -> (39, -13.3431)
  line L1858 (39, -13.3431) -> (39, -16.6569)
  line L1859 (39, -16.6569) -> (36.6569, -19)
  line L1860 (36.6569, -19) -> (33.3431, -19)
  line L1861 (33.3431, -19) -> (31, -16.6569)
  line L1862 (41, -26.6569) -> (41, -23.3431)
  line L1863 (41, -23.3431) -> (43.3431, -21)
  line L1864 (43.3431, -21) -> (46.6569, -21)
  line L1865 (46.6569, -21) -> (49, -23.3431)
  line L1866 (49, -23.3431) -> (49, -26.6569)
  line L1867 (49, -26.6569) -> (46.6569, -29)
  line L1868 (46.6569, -29) -> (43.3431, -29)
  line L1869 (43.3431, -29) -> (41, -26.6569)
  line L1870 (1, -16.6569) -> (1, -13.3431)
  line L1871 (1, -13.3431) -> (3.3431, -11)
  line L1872 (3.3431, -11) -> (6.6569, -11)
  line L1873 (6.6569, -11) -> (9, -13.3431)
  line L1874 (9, -13.3431) -> (9, -16.6569)
  line L1875 (9, -16.6569) -> (6.6569, -19)
  line L1876 (6.6569, -19) -> (3.3431, -19)
  line L1877 (3.3431, -19) -> (1, -16.6569)
  line L1878 (11, -16.6569) -> (11, -13.3431)
  line L1879 (11, -13.3431) -> (13.3431, -11)
  line L1880 (13.3431, -11) -> (16.6569, -11)
  line L1881 (16.6569, -11) -> (19, -13.3431)
  line L1882 (19, -13.3431) -> (19, -16.6569)
  line L1883 (19, -16.6569) -> (16.6569, -19)
  line L1884 (16.6569, -19) -> (13.3431, -19)
  line L1885 (13.3431, -19) -> (11, -16.6569)
  line L1886 (-19, -16.6569) -> (-19, -13.3431)
  line L1887 (-19, -13.3431) -> (-16.6569, -11)
  line L1888 (-16.6569, -11) -> (-13.3431, -11)
  line L1889 (-13.3431, -11) -> (-11, -13.3431)
  line L1890 (-11, -13.3431) -> (-11, -16.6569)
  line L1891 (-11, -16.6569) -> (-13.3431, -19)
  line L1892 (-13.3431, -19) -> (-16.6569, -19)
  line L1893 (-16.6569, -19) -> (-19, -16.6569)
  line L1894 (-39, -16.6569) -> (-39, -13.3431)
  line L1895 (-39, -13.3431) -> (-36.6569, -11)
  line L1896 (-36.6569, -11) -> (-33.3431, -11)
  line L1897 (-33.3431, -11) -> (-31, -13.3431)
  line L1898 (-31, -13.3431) -> (-31, -16.6569)
  line L1899 (-31, -16.6569) -> (-33.3431, -19)
  line L1900 (-33.3431, -19) -> (-36.6569, -19)
  line L1901 (-36.6569, -19) -> (-39, -16.6569)
  line L1902 (61, -26.6569) -> (61, -23.3431)
  line L1903 (61, -23.3431) -> (63.3431, -21)
  line L1904 (63.3431, -21) -> (66.6569, -21)
  line L1905 (66.6569, -21) -> (69, -23.3431)
  line L1906 (69, -23.3431) -> (69, -26.6569)
  line L1907 (69, -26.6569) -> (66.6569, -29)
  line L1908 (66.6569, -29) -> (63.3431, -29)
  line L1909 (63.3431, -29) -> (61, -26.6569)
  line L1910 (1, 53.3431) -> (1, 56.6569)
  line L1911 (1, 56.6569) -> (3.3431, 59)
  line L1912 (3.3431, 59) -> (6.6569, 59)
  line L1913 (6.6569, 59) -> (9, 56.6569)
  line L1914 (9, 56.6569) -> (9, 53.3431)
  line L1915 (9, 53.3431) -> (6.6569, 51)
  line L1916 (6.6569, 51) -> (3.3431, 51)
  line L1917 (3.3431, 51) -> (1, 53.3431)
  line L1918 (11, 53.3431) -> (11, 56.6569)
  line L1919 (11, 56.6569) -> (13.3431, 59)
  line L1920 (13.3431, 59) -> (16.6569, 59)
  line L1921 (16.6569, 59) -> (19, 56.6569)
  line L1922 (19, 56.6569) -> (19, 53.3431)
  line L1923 (19, 53.3431) -> (16.6569, 51)
  line L1924 (16.6569, 51) -> (13.3431, 51)
  line L1925 (13.3431, 51) -> (11, 53.3431)
  line L1926 (31, 53.3431) -> (31, 56.6569)
  line L1927 (31, 56.6569) -> (33.3431, 59)
  line L1928 (33.3431, 59) -> (36.6569, 59)
  line L1929 (36.6569, 59) -> (39, 56.6569)
  line L1930 (39, 56.6569) -> (39, 53.3431)
  line L1931 (39, 53.3431) -> (36.6569, 51)
  line L1932 (36.6569, 51) -> (33.3431, 51)
  line L1933 (33.3431, 51) -> (31, 53.3431)
  line L1934 (21, 53.3431) -> (21, 56.6569)
  line L1935 (21, 56.6569) -> (23.3431, 59)
  line L1936 (23.3431, 59) -> (26.6569, 59)
  line L1937 (26.6569, 59) -> (29, 56.6569)
  line L1938 (29, 56.6569) -> (29, 53.3431)
  line L1939 (29, 53.3431) -> (26.6569, 51)
  line L1940 (26.6569, 51) -> (23.3431, 51)
  line L1941 (23.3431, 51) -> (21, 53.3431)
  line L1942 (61, 53.3431) -> (61, 56.6569)
  line L1943 (61, 56.6569) -> (63.3431, 59)
  line L1944 (63.3431, 59) -> (66.6569, 59)
  line L1945 (66.6569, 59) -> (69, 56.6569)
  line L1946 (69, 56.6569) -> (69, 53.3431)
  line L1947 (69, 53.3431) -> (66.6569, 51)
  line L1948 (66.6569, 51) -> (63.3431, 51)
  line L1949 (63.3431, 51) -> (61, 53.3431)
  line L1950 (-9, 53.3431) -> (-9, 56.6569)
  line L1951 (-9, 56.6569) -> (-6.6569, 59)
  line L1952 (-6.6569, 59) -> (-3.3431, 59)
  line L1953 (-3.3431, 59) -> (-1, 56.6569)
  line L1954 (-1, 56.6569) -> (-1, 53.3431)
  line L1955 (-1, 53.3431) -> (-3.3431, 51)
  line L1956 (-3.3431, 51) -> (-6.6569, 51)
  line L1957 (-6.6569, 51) -> (-9, 53.3431)
  line L1958 (-69, 63.3431) -> (-69, 66.6569)
  line L1959 (-69, 66.6569) -> (-66.6569, 69)
  line L1960 (-66.6569, 69) -> (-63.3431, 69)
  line L1961 (-63.3431, 69) -> (-61, 66.6569)
  line L1962 (-61, 66.6569) -> (-61, 63.3431)
  line L1963 (-61, 63.3431) -> (-63.3431, 61)
  line L1964 (-63.3431, 61) -> (-66.6569, 61)
  line L1965 (-66.6569, 61) -> (-69, 63.3431)
  line L1966 (-19, 53.3431) -> (-19, 56.6569)
  line L1967 (-19, 56.6569) -> (-16.6569, 59)
  line L1968 (-16.6569, 59) -> (-13.3431, 59)
  line L1969 (-13.3431, 59) -> (-11, 56.6569)
  line L1970 (-11, 56.6569) -> (-11, 53.3431)
  line L1971 (-11, 53.3431) -> (-13.3431, 51)
  line L1972 (-13.3431, 51) -> (-16.6569, 51)
  line L1973 (-16.6569, 51) -> (-19, 53.3431)
  line L1974 (-29, 53.3431) -> (-29, 56.6569)
  line L1975 (-29, 56.6569) -> (-26.6569, 59)
  line L1976 (-26.6569, 59) -> (-23.3431, 59)
  line L1977 (-23.3431, 59) -> (-21, 56.6569)
  line L1978 (-21, 56.6569) -> (-21, 53.3431)
  line L1979 (-21, 53.3431) -> (-23.3431, 51)
  line L1980 (-23.3431, 51) -> (-26.6569, 51)
  line L1981 (-26.6569, 51) -> (-29, 53.3431)
  line L1982 (-39, 53.3431) -> (-39, 56.6569)
  line L1983 (-39, 56.6569) -> (-36.6569, 59)
  line L1984 (-36.6569, 59) -> (-33.3431, 59)
  line L1985 (-33.3431, 59) -> (-31, 56.6569)
  line L1986 (-31, 56.6569) -> (-31, 53.3431)
  line L1987 (-31, 53.3431) -> (-33.3431, 51)
  line L1988 (-33.3431, 51) -> (-36.6569, 51)
  line L1989 (-36.6569, 51) -> (-39, 53.3431)
  line L1990 (-49, 53.3431) -> (-49, 56.6569)
  line L1991 (-49, 56.6569) -> (-46.6569, 59)
  line L1992 (-46.6569, 59) -> (-43.3431, 59)
  line L1993 (-43.3431, 59) -> (-41, 56.6569)
  line L1994 (-41, 56.6569) -> (-41, 53.3431)
  line L1995 (-41, 53.3431) -> (-43.3431, 51)
  line L1996 (-43.3431, 51) -> (-46.6569, 51)
  line L1997 (-46.6569, 51) -> (-49, 53.3431)
  line L1998 (-59, 53.3431) -> (-59, 56.6569)
  line L1999 (-59, 56.6569) -> (-56.6569, 59)
  line L2000 (-56.6569, 59) -> (-53.3431, 59)
  line L2001 (-53.3431, 59) -> (-51, 56.6569)
  line L2002 (-51, 56.6569) -> (-51, 53.3431)
  line L2003 (-51, 53.3431) -> (-53.3431, 51)
  line L2004 (-53.3431, 51) -> (-56.6569, 51)
  line L2005 (-56.6569, 51) -> (-59, 53.3431)
  line L2006 (-69, 53.3431) -> (-69, 56.6569)
  line L2007 (-69, 56.6569) -> (-66.6569, 59)
  line L2008 (-66.6569, 59) -> (-63.3431, 59)
  line L2009 (-63.3431, 59) -> (-61, 56.6569)
  line L2010 (-61, 56.6569) -> (-61, 53.3431)
  line L2011 (-61, 53.3431) -> (-63.3431, 51)
  line L2012 (-63.3431, 51) -> (-66.6569, 51)
  line L2013 (-66.6569, 51) -> (-69, 53.3431)
  line L2014 (61, 43.3431) -> (61, 46.6569)
  line L2015 (61, 46.6569) -> (63.3431, 49)
  line L2016 (63.3431, 49) -> (66.6569, 49)
  line L2017 (66.6569, 49) -> (69, 46.6569)
  line L2018 (69, 46.6569) -> (69, 43.3431)
  line L2019 (69, 43.3431) -> (66.6569, 41)
  line L2020 (66.6569, 41) -> (63.3431, 41)
  line L2021 (63.3431, 41) -> (61, 43.3431)
  line L2022 (51, 43.3431) -> (51, 46.6569)
  line L2023 (51, 46.6569) -> (53.3431, 49)
  line L2024 (53.3431, 49) -> (56.6569, 49)
  line L2025 (56.6569, 49) -> (59, 46.6569)
  line L2026 (59, 46.6569) -> (59, 43.3431)
  line L2027 (59, 43.3431) -> (56.6569, 41)
  line L2028 (56.6569, 41) -> (53.3431, 41)
  line L2029 (53.3431, 41) -> (51, 43.3431)
  line L2030 (41, 43.3431) -> (41, 46.6569)
  line L2031 (41, 46.6569) -> (43.3431, 49)
  line L2032 (43.3431, 49) -> (46.6569, 49)
  line L2033 (46.6569, 49) -> (49, 46.6569)
  line L2034 (49, 46.6569) -> (49, 43.3431)
  line L2035 (49, 43.3431) -> (46.6569, 41)
  line L2036 (46.6569, 41) -> (43.3431, 41)
  line L2037 (43.3431, 41) -> (41, 43.3431)
  line L2038 (31, 43.3431) -> (31, 46.6569)
  line L2039 (31, 46.6569) -> (33.3431, 49)
  line L2040 (33.3431, 49) -> (36.6569, 49)
  line L2041 (36.6569, 49) -> (39, 46.6569)
  line L2042 (39, 46.6569) -> (39, 43.3431)
  line L2043 (39, 43.3431) -> (36.6569, 41)
  line L2044 (36.6569, 41) -> (33.3431, 41)
  line L2045 (33.3431, 41) -> (31, 43.3431)
  line L2046 (51, 53.3431) -> (51, 56.6569)
  line L2047 (51, 56.6569) -> (53.3431, 59)
  line L2048 (53.3431, 59) -> (56.6569, 59)
  line L2049 (56.6569, 59) -> (59, 56.6569)
  line L2050 (59, 56.6569) -> (59, 53.3431)
  line L2051 (59, 53.3431) -> (56.6569, 51)
  line L2052 (56.6569, 51) -> (53.3431, 51)
  line L2053 (53.3431, 51) -> (51, 53.3431)
  line L2054 (41, 53.3431) -> (41, 56.6569)
  line L2055 (41, 56.6569) -> (43.3431, 59)
  line L2056 (43.3431, 59) -> (46.6569, 59)
  line L2057 (46.6569, 59) -> (49, 56.6569)
  line L2058 (49, 56.6569) -> (49, 53.3431)
  line L2059 (49, 53.3431) -> (46.6569, 51)
  line L2060 (46.6569, 51) -> (43.3431, 51)
  line L2061 (43.3431, 51) -> (41, 53.3431)
  line L2062 (-59, 63.3431) -> (-59, 66.6569)
  line L2063 (-59, 66.6569) -> (-56.6569, 69)
  line L2064 (-56.6569, 69) -> (-53.3431, 69)
  line L2065 (-53.3431, 69) -> (-51, 66.6569)
  line L2066 (-51, 66.6569) -> (-51, 63.3431)
  line L2067 (-51, 63.3431) -> (-53.3431, 61)
  line L2068 (-53.3431, 61) -> (-56.6569, 61)
  line L2069 (-56.6569, 61) -> (-59, 63.3431)
  line L2070 (41, 13.3431) -> (41, 16.6569)
  line L2071 (41, 16.6569) -> (43.3431, 19)
  line L2072 (43.3431, 19) -> (46.6569, 19)
  line L2073 (46.6569, 19) -> (49, 16.6569)
  line L2074 (49, 16.6569) -> (49, 13.3431)
  line L2075 (49, 13.3431) -> (46.6569, 11)
  line L2076 (46.6569, 11) -> (43.3431, 11)
  line L2077 (43.3431, 11) -> (41, 13.3431)
  line L2078 (51, 13.3431) -> (51, 16.6569)
  line L2079 (51, 16.6569) -> (53.3431, 19)
  line L2080 (53.3431, 19) -> (56.6569, 19)
  line L2081 (56.6569, 19) -> (59, 16.6569)
  line L2082 (59, 16.6569) -> (59, 13.3431)
  line L2083 (59, 13.3431) -> (56.6569, 11)
  line L2084 (56.6569, 11) -> (53.3431, 11)
  line L2085 (53.3431, 11) -> (51, 13.3431)
  line L2086 (61, 13.3431) -> (61, 16.6569)
  line L2087 (61, 16.6569) -> (63.3431, 19)
  line L2088 (63.3431, 19) -> (66.6569, 19)
  line L2089 (66.6569, 19) -> (69, 16.6569)
  line L2090 (69, 16.6569) -> (69, 13.3431)
  line L2091 (69, 13.3431) -> (66.6569, 11)
  line L2092 (66.6569, 11) -> (63.3431, 11)
  line L2093 (63.3431, 11) -> (61, 13.3431)
  line L2094 (-69, 23.3431) -> (-69, 26.6569)
  line L2095 (-69, 26.6569) -> (-66.6569, 29)
  line L2096 (-66.6569, 29) -> (-63.3431, 29)
  line L2097 (-63.3431, 29) -> (-61, 26.6569)
  line L2098 (-61, 26.6569) -> (-61, 23.3431)
  line L2099 (-61, 23.3431) -> (-63.3431, 21)
  line L2100 (-63.3431, 21) -> (-66.6569, 21)
  line L2101 (-66.6569, 21) -> (-69, 23.3431)
  line L2102 (-59, 23.3431) -> (-59, 26.6569)
  line L2103 (-59, 26.6569) -> (-56.6569, 29)
  line L2104 (-56.6569, 29) -> (-53.3431, 29)
  line L2105 (-53.3431, 29) -> (-51, 26.6569)
  line L2106 (-51, 26.6569) -> (-51, 23.3431)
  line L2107 (-51, 23.3431) -> (-53.3431, 21)
  line L2108 (-53.3431, 21) -> (-56.6569, 21)
  line L2109 (-56.6569, 21) -> (-59, 23.3431)
  line L2110 (-49, 23.3431) -> (-49, 26.6569)
  line L2111 (-49, 26.6569) -> (-46.6569, 29)
  line L2112 (-46.6569, 29) -> (-43.3431, 29)
  line L2113 (-43.3431, 29) -> (-41, 26.6569)
  line L2114 (-41, 26.6569) -> (-41, 23.3431)
  line L2115 (-41, 23.3431) -> (-43.3431, 21)
  line L2116 (-43.3431, 21) -> (-46.6569, 21)
  line L2117 (-46.6569, 21) -> (-49, 23.3431)
  line L2118 (-39, 23.3431) -> (-39, 26.6569)
  line L2119 (-39, 26.6569) -> (-36.6569, 29)
  line L2120 (-36.6569, 29) -> (-33.3431, 29)
  line L2121 (-33.3431, 29) -> (-31, 26.6569)
  line L2122 (-31, 26.6569) -> (-31, 23.3431)
  line L2123 (-31, 23.3431) -> (-33.3431, 21)
  line L2124 (-33.3431, 21) -> (-36.6569, 21)
  line L2125 (-36.6569, 21) -> (-39, 23.3431)
  line L2126 (-29, 23.3431) -> (-29, 26.6569)
  line L2127 (-29, 26.6569) -> (-26.6569, 29)
  line L2128 (-26.6569, 29) -> (-23.3431, 29)
  line L2129 (-23.3431, 29) -> (-21, 26.6569)
  line L2130 (-21, 26.6569) -> (-21, 23.3431)
  line L2131 (-21, 23.3431) -> (-23.3431, 21)
  line L2132 (-23.3431, 21) -> (-26.6569, 21)
  line L2133 (-26.6569, 21) -> (-29, 23.3431)
  line L2134 (-19, 23.3431) -> (-19, 26.6569)
  line L2135 (-19, 26.6569) -> (-16.6569, 29)
  line L2136 (-16.6569, 29) -> (-13.3431, 29)
  line L2137 (-13.3431, 29) -> (-11, 26.6569)
  line L2138 (-11, 26.6569) -> (-11, 23.3431)
  line L2139 (-11, 23.3431) -> (-13.3431, 21)
  line L2140 (-13.3431, 21) -> (-16.6569, 21)
  line L2141 (-16.6569, 21) -> (-19, 23.3431)
  line L2142 (-9, 23.3431) -> (-9, 26.6569)
  line L2143 (-9, 26.6569) -> (-6.6569, 29)
  line L2144 (-6.6569, 29) -> (-3.3431, 29)
  line L2145 (-3.3431, 29) -> (-1, 26.6569)
  line L2146 (-1, 26.6569) -> (-1, 23.3431)
  line L2147 (-1, 23.3431) -> (-3.3431, 21)
  line L2148 (-3.3431, 21) -> (-6.6569, 21)
  line L2149 (-6.6569, 21) -> (-9, 23.3431)
  line L2150 (1, 23.3431) -> (1, 26.6569)
  line L2151 (1, 26.6569) -> (3.3431, 29)
  line L2152 (3.3431, 29) -> (6.6569, 29)
  line L2153 (6.6569, 29) -> (9, 26.6569)
  line L2154 (9, 26.6569) -> (9, 23.3431)
  line L2155 (9, 23.3431) -> (6.6569, 21)
  line L2156 (6.6569, 21) -> (3.3431, 21)
  line L2157 (3.3431, 21) -> (1, 23.3431)
  line L2158 (11, 23.3431) -> (11, 26.6569)
  line L2159 (11, 26.6569) -> (13.3431, 29)
  line L2160 (13.3431, 29) -> (16.6569, 29)
  line L2161 (16.6569, 29) -> (19, 26.6569)
  line L2162 (19, 26.6569) -> (19, 23.3431)
  line L2163 (19, 23.3431) -> (16.6569, 21)
  line L2164 (16.6569, 21) -> (13.3431, 21)
  line L2165 (13.3431, 21) -> (11, 23.3431)
  line L2166 (21, 23.3431) -> (21, 26.6569)
  line L2167 (21, 26.6569) -> (23.3431, 29)
  line L2168 (23.3431, 29) -> (26.6569, 29)
  line L2169 (26.6569, 29) -> (29, 26.6569)
  line L2170 (29, 26.6569) -> (29, 23.3431)
  line L2171 (29, 23.3431) -> (26.6569, 21)
  line L2172 (26.6569, 21) -> (23.3431, 21)
  line L2173 (23.3431, 21) -> (21, 23.3431)
  line L2174 (31, 23.3431) -> (31, 26.6569)
  line L2175 (31, 26.6569) -> (33.3431, 29)
  line L2176 (33.3431, 29) -> (36.6569, 29)
  line L2177 (36.6569, 29) -> (39, 26.6569)
  line L2178 (39, 26.6569) -> (39, 23.3431)
  line L2179 (39, 23.3431) -> (36.6569, 21)
  line L2180 (36.6569, 21) -> (33.3431, 21)
  line L2181 (33.3431, 21) -> (31, 23.3431)
  line L2182 (41, 23.3431) -> (41, 26.6569)
  line L2183 (41, 26.6569) -> (43.3431, 29)
  line L2184 (43.3431, 29) -> (46.6569, 29)
  line L2185 (46.6569, 29) -> (49, 26.6569)
  line L2186 (49, 26.6569) -> (49, 23.3431)
  line L2187 (49, 23.3431) -> (46.6569, 21)
  line L2188 (46.6569, 21) -> (43.3431, 21)
  line L2189 (43.3431, 21) -> (41, 23.3431)
  line L2190 (51, 23.3431) -> (51, 26.6569)
  line L2191 (51, 26.6569) -> (53.3431, 29)
  line L2192 (53.3431, 29) -> (56.6569, 29)
  line L2193 (56.6569, 29) -> (59, 26.6569)
  line L2194 (59, 26.6569) -> (59, 23.3431)
  line L2195 (59, 23.3431) -> (56.6569, 21)
  line L2196 (56.6569, 21) -> (53.3431, 21)
  line L2197 (53.3431, 21) -> (51, 23.3431)
  line L2198 (61, 23.3431) -> (61, 26.6569)
  line L2199 (61, 26.6569) -> (63.3431, 29)
  line L2200 (63.3431, 29) -> (66.6569, 29)
  line L2201 (66.6569, 29) -> (69, 26.6569)
  line L2202 (69, 26.6569) -> (69, 23.3431)
  line L2203 (69, 23.3431) -> (66.6569, 21)
  line L2204 (66.6569, 21) -> (63.3431, 21)
  line L2205 (63.3431, 21) -> (61, 23.3431)
  line L2206 (-69, 33.3431) -> (-69, 36.6569)
  line L2207 (-69, 36.6569) -> (-66.6569, 39)
  line L2208 (-66.6569, 39) -> (-63.3431, 39)
  line L2209 (-63.3431, 39) -> (-61, 36.6569)
  line L2210 (-61, 36.6569) -> (-61, 33.3431)
  line L2211 (-61, 33.3431) -> (-63.3431, 31)
  line L2212 (-63.3431, 31) -> (-66.6569, 31)
  line L2213 (-66.6569, 31) -> (-69, 33.3431)
  line L2214 (-59, 33.3431) -> (-59, 36.6569)
  line L2215 (-59, 36.6569) -> (-56.6569, 39)
  line L2216 (-56.6569, 39) -> (-53.3431, 39)